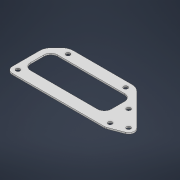
# Autodesk Inventor part: gusset-2-3.25-full-no-front
Saved by Autodesk Inventor 2021 (Build 250183000, 183)
## iProperties
Created: 2020-11-04
Part Number: gusset-2-3.25-full-no-front
Material: Generic
Document SubType Name: Modeling
Designer: Carlos Stewart
Density: 1 g/cm^3
Appearance: Default
Author: Carlos Stewart
Autodesk Inventor part; units mm, degrees
ref_plane "YZ Plane" through (0, 0, 0) normal (1, 0, 0) x (0, 1, 0)
ref_plane "XZ Plane" through (0, 0, 0) normal (0, 1, 0) x (-1, 0, 0)
ref_plane "XY Plane" through (0, 0, 0) normal (0, 0, 1) x (1, 0, 0)
sketch "Sketch1" plane through (0, 0, 0) normal (0, 1, 0) x (-1, 0, 0)
  line L0 (-37.8542, -1.1176) -> (35.8058, -1.1176)
  line L1 (43.4258, -8.7376) -> (43.4258, -23.2918)
  line L2 (35.8058, -30.9118) -> (-37.8542, -30.9118)
  line L3 (-45.4742, -23.2918) -> (-45.4742, -8.7376)
  arc A0 (-37.8542, -1.1176) -> (-45.4742, -8.7376) centre (-37.8542, -8.7376) ccw
  arc A1 (-45.4742, -23.2918) -> (-37.8542, -30.9118) centre (-37.8542, -23.2918) ccw
  arc A2 (35.8058, -30.9118) -> (43.4258, -23.2918) centre (35.8058, -23.2918) ccw
  arc A3 (43.4258, -8.7376) -> (35.8058, -1.1176) centre (35.8058, -8.7376) ccw
  circle A4 centre (-72.8662, -0.3634) radius 2.3114
  circle A5 centre (-54.9057, -18.324) radius 2.3114
  circle A6 centre (-58.1742, 5.2324) radius 2.3114
  circle A7 centre (-32.7742, -37.2618) radius 2.3114
  circle A8 centre (30.7258, -37.2618) radius 2.3114
  circle A9 centre (43.4258, 5.2324) radius 2.3114
  arc A10 (49.7758, 5.2324) -> (43.4258, 11.5824) centre (43.4258, 5.2324) ccw
  arc A11 (-75.1264, 5.5707) -> (-77.3564, -4.8536) centre (-72.8662, -0.3634) ccw
  arc A12 (-58.1742, 11.5824) -> (-60.4344, 11.1665) centre (-58.1742, 5.2324) ccw
  line L4 (35.8058, -30.9118) -> (-37.8542, -30.9118)
  line L5 (-75.1264, 5.5707) -> (-60.4344, 11.1665)
  line L6 (-77.3564, -4.8536) -> (-42.3179, -39.8921)
  line L7 (-33.3376, -43.6118) -> (31.2893, -43.6118)
  line L8 (-58.1742, 11.5824) -> (43.4258, 11.5824)
  arc A13 (-42.3179, -39.8921) -> (-33.3376, -43.6118) centre (-33.3376, -30.9118) ccw
  arc A14 (35.8058, -30.9118) -> (43.4258, -23.2918) centre (35.8058, -23.2918) ccw
  line L9 (46.0561, -34.1055) -> (40.2695, -39.8921)
  arc A15 (31.2893, -43.6118) -> (40.2695, -39.8921) centre (31.2893, -30.9118) ccw
  line L10 (49.7758, 5.2324) -> (49.7758, -25.1252)
  arc A16 (46.0561, -34.1055) -> (49.7758, -25.1252) centre (37.0758, -25.1252) ccw
  point P0 (0, 0)
  point P1 (43.4258, -30.9118)
  point P2 (43.4258, -1.1176)
  point P3 (-45.4742, -30.9118)
  point P4 (43.4258, -30.9118)
  point P5 (41.194, -28.68)
  dimension "d2" = 7.62
  dimension "d21" = 12.7
  constraints: 23 point on circle, 23 tangent, 22 end point, 17 centre point, 6 point on line, 4 coincident, 3 equal radius, 2 horizontal, 2 parallel, 1 perpendicular, 1 vertical, 10 other
  measures "d2" radius of A0
  measures "d21" radius of A13
extrude "Extrusion1" add sketch "Sketch1" along normal blind 1.5875
body "Solid1"
